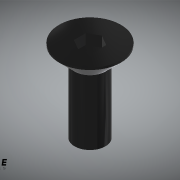
# Autodesk Inventor part: ねじ皿　m3-l8
Saved by Autodesk Inventor 2020 (Build 240168000, 168)
## iProperties
Created: 2017-02-12
Part Number: ねじ皿　m3-l8
Material: 鋼
Document SubType Name: Modeling
Designer: 大空
Mass: 0.560984 g
Surface Area: 1.35407 cm^2
Volume: 0.0714629 cm^3
Density: 7.85 g/cm^3
Appearance: 滑らか - 黒
Author: 大空
Autodesk Inventor part; units mm, degrees
ref_plane "YZ Plane" through (0, 0, 0) normal (1, 0, 0) x (0, 1, 0)
ref_plane "XZ Plane" through (0, 0, 0) normal (0, 1, 0) x (-1, 0, 0)
ref_plane "XY Plane" through (0, 0, 0) normal (0, 0, 1) x (1, 0, 0)
sketch "スケッチ1" plane through (0, 0, 0) normal (0, 0, 1) x (1, 0, 0)
  circle A0 centre (0, 0) radius 1.5
  dimension "d0" = 3
  constraints: 1 centre point, 1 coincident
  measures "d0" diameter of A0
extrude "押し出し1" add sketch "スケッチ1" along normal blind 8
sketch "スケッチ2" plane through (0, 0, 8) normal (0, 0, 1) x (1, 0, 0)
  circle A0 centre (0, 0) radius 1.5 projected
  circle A1 centre (0, 0) radius 3
  line L0 (0, 1.1547) -> (1, 0.5774)
  line L1 (1, 0.5774) -> (1, -0.5774)
  line L2 (1, -0.5774) -> (0, -1.1547)
  line L3 (0, -1.1547) -> (-1, -0.5774)
  line L4 (-1, -0.5774) -> (-1, 0.5774)
  line L5 (-1, 0.5774) -> (0, 1.1547)
  dimension "d3" = 6
  dimension "d6" = 2
  constraints: 12 end point, 2 coincident, 1 centre point, 1 vertical, 13 other
  measures "d3" diameter of A1
  measures "d6" distance between parallel lines of L1 L4
extrude "押し出し2" add sketch "スケッチ2" against normal blind 1.7 contours A1
extrude "押し出し3" cut sketch "スケッチ2" against normal blind 1 contours L0 L1 L2 L3 L4 L5
chamfer "面取り1" distance 1.5 angle 45 1 edges at (-3, 0, 6.3)
